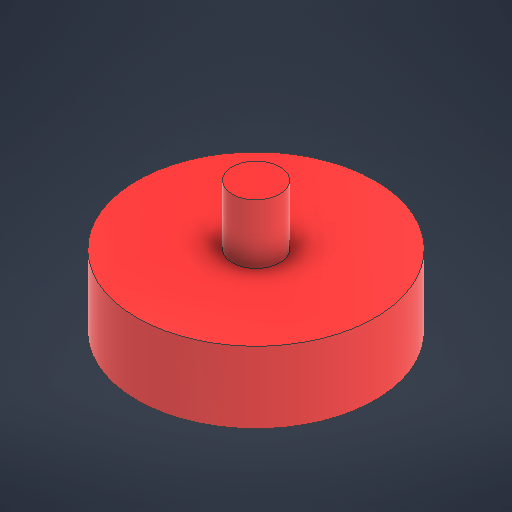
# Autodesk Inventor part: Prindere_aux
Saved by Autodesk Inventor 2026.1 (Build 301233000, 233)
## iProperties
Created: 2025-08-25
Part Number: Prindere_aux
Material: Generic
Document SubType Name: Modeling
Designer: emanuel
Density: 1 g/cm^3
Appearance: Default
Author: emanuel
Autodesk Inventor part; units mm, degrees
ref_plane "YZ Plane" through (0, 0, 0) normal (1, 0, 0) x (0, 1, 0)
ref_plane "XZ Plane" through (0, 0, 0) normal (0, 1, 0) x (-1, 0, 0)
ref_plane "XY Plane" through (0, 0, 0) normal (0, 0, 1) x (1, 0, 0)
sketch "Sketch1" plane through (0, 0, 0) normal (1, 0, 0) x (0, 1, 0)
  line L0 (0, 0) -> (8, 0)
  line L1 (0, 0) -> (6, 0)
  line L2 (6, 0) -> (6, -10)
  line L3 (6, -10) -> (0, -10)
  line L4 (0, -10) -> (0, 0)
  line L5 (6, 0) -> (11, 0)
  line L6 (11, 0) -> (11, -2)
  line L7 (11, -2) -> (6, -2)
  line L8 (6, -2) -> (6, 0)
  dimension "d0" = 8
  dimension "d1" = 6
  dimension "d2" = 10
  dimension "d3" = 5
  dimension "d4" = 2
  constraints: 18 end point, 4 parallel, 3 horizontal, 2 perpendicular
  measures "d0" distance of L0.start L0.end
  measures "d1" distance of L2.end L3.end
  measures "d2" distance of L1.end L2.end
  measures "d3" distance of L6.end L7.end
  measures "d4" distance of L5.end L6.end
revolve "Revolution1" add sketch "Sketch1" angle 360 about axis through (0, 0, 0) along (0, 1, 0)
body "Solid1"
